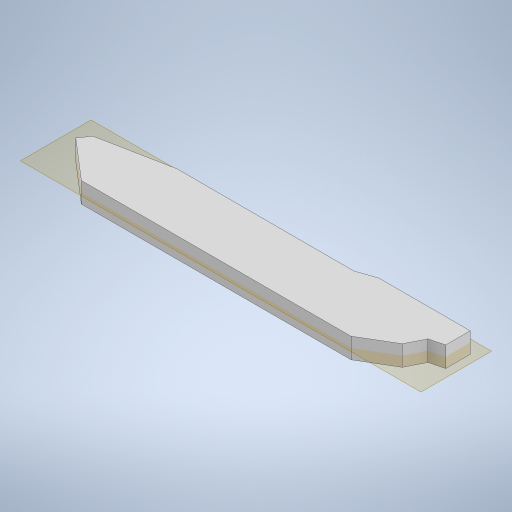
# Autodesk Inventor part: Friend_track_collision
Saved by Autodesk Inventor 2024 (Build 280153000, 153)
## iProperties
Created: 2026-05-25
Part Number: Friend_track_collision
Material: Generic
Document SubType Name: Modeling
Designer: warny
Density: 1 g/cm^3
Appearance: Default
Author: warny
Autodesk Inventor part; units mm, degrees
ref_plane "YZ Plane" through (0, 0, 0) normal (1, 0, 0) x (0, 1, 0)
ref_plane "XY Plane" through (0, 0, 0) normal (0, 0, 1) x (1, 0, 0)
sketch "Sketch1" plane through (0, 0, 0) normal (0, 1, 0) x (-1, 0, 0)
  line L0 (0, -144.8636) -> (0, 84.5516) construction
  line L1 (624.86, 0) -> (-675.46, 0) construction
  line L2 (338.2, 51.778) -> (439.1, -35.05)
  line L3 (439.1, -35.05) -> (421.2, -60.89)
  line L4 (421.2, -60.89) -> (242.5, -95.89)
  line L5 (242.5, -95.89) -> (-209.7, -95.89)
  line L6 (-209.7, -95.89) -> (-256.7, -112.09)
  line L7 (-256.7, -112.09) -> (-489.7, -112.09)
  line L8 (-489.7, -112.09) -> (-489.7, -49.69)
  line L9 (-489.7, -49.69) -> (-453.7, -40.3)
  line L10 (-453.7, -40.3) -> (-431.7, 3.13)
  line L11 (-431.7, 3.13) -> (-349.7, 51.778)
  line L12 (-349.7, 51.778) -> (338.2, 51.778)
  point P0 (0, 0)
  dimension "d0" = 51.778
  dimension "d1" = 35.05
  dimension "d2" = 60.89
  dimension "d3" = 95.89
  dimension "d4" = 95.89
  dimension "d5" = 112.09
  dimension "d6" = 112.09
  dimension "d8" = 40.3
  dimension "d9" = 49.69
  dimension "d10" = 3.13
  dimension "d11" = 51.778
  dimension "d12" = 338.2
  dimension "d13" = 439.1
  dimension "d14" = 421.2
  dimension "d15" = 242.5
  dimension "d16" = 489.7
  dimension "d17" = 256.7
  dimension "d18" = 209.7
  dimension "d19" = 489.7
  dimension "d20" = 453.7
  dimension "d21" = 431.7
  dimension "d22" = 349.7
  constraints: 22 end point
  measures "d0" distance from line of L2.start L1
  measures "d1" distance from line of L1 L2.end
  measures "d2" distance from line of L1 L3.end
  measures "d3" distance from line of L1 L4.end
  measures "d4" distance from line of L1 L5.end
  measures "d5" distance from line of L1 L6.end
  measures "d6" distance from line of L1 L7.end
  measures "d8" distance from line of L1 L9.end
  measures "d9" distance from line of L1 L8.end
  measures "d10" distance from line of L1 L10.end
  measures "d11" distance from line of L1 L11.end
  measures "d12" distance from line of L2.start L0
  measures "d13" distance from line of L0 L2.end
  measures "d14" distance from line of L0 L3.end
  measures "d15" distance from line of L0 L4.end
  measures "d16" distance from line of L0 L7.end
  measures "d17" distance from line of L0 L6.end
  measures "d18" distance from line of L0 L5.end
  measures "d19" distance from line of L0 L8.end
  measures "d20" distance from line of L0 L9.end
  measures "d21" distance from line of L0 L10.end
  measures "d22" distance from line of L0 L11.end
extrude "Extrusion1" add sketch "Sketch1" along normal mid plane 52
body "Solid1"
